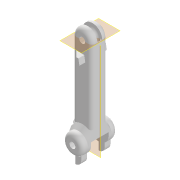
# Autodesk Inventor part: index_f1
Saved by Autodesk Inventor 2020.2 (Build 242310000, 310)
## iProperties
Created: 2020-04-08
Part Number: index_f1
Material: Generic
Document SubType Name: Modeling
Designer: Bardo91
Density: 1 g/cm^3
Appearance: Default
Author: Bardo91
Autodesk Inventor part; units mm, degrees
ref_plane "YZ Plane" through (0, 0, 0) normal (1, 0, 0) x (0, 1, 0)
ref_plane "XY Plane" through (0, 0, 0) normal (0, 0, 1) x (1, 0, 0)
sketch "Sketch1" plane through (0, 0, 0) normal (0, 0, 1) x (1, 0, 0)
  circle A0 centre (0, 0) radius 1.5
  line L0 (0, 0) -> (0, 44)
  circle A1 centre (0, 44) radius 1.5
  circle A2 centre (0, 44) radius 5
  circle A3 centre (0, 0) radius 5
  line L1 (-5, 44) -> (-5, 0)
  line L2 (5, 0) -> (5, 44)
  point P0 (0, 39)
  point P1 (0, 5)
  dimension "d0" = 3
  dimension "d1" = 44
  dimension "d2" = 3
  dimension "d3" = 10
  dimension "d4" = 10
  constraints: 6 end point, 4 centre point, 4 coincident, 4 point on circle, 2 tangent, 2 vertical
  measures "d0" diameter of A0
  measures "d1" distance of L0.start L0.end
  measures "d2" diameter of A1
  measures "d3" diameter of A2
  measures "d4" diameter of A3
extrude "base" add sketch "Sketch1" along normal blind 8
sketch "Sketch2" plane through (0, 0, 8) normal (0, 0, 1) x (1, 0, 0)
  circle A0 centre (0, 0) radius 1.5 projected
  circle A1 centre (0, 0) radius 5
  circle A2 centre (0, 0) radius 1.5
  dimension "d7" = 10
  dimension "d8" = 3
  constraints: 2 centre point, 2 coincident
  measures "d7" diameter of A1
  measures "d8" diameter of A2
extrude "joint" add sketch "Sketch2" along normal blind 5
ref_plane "Work Plane1" through (0, 0, 4) normal (0, 0, 1) x (1, 0, 0)
mirror "Mirror1" about plane through (0, 0, 4) normal (0, 0, 1) of "joint"
chamfer "Chamfer1" distance 2 angle 45 2 edges at (0, 5, 8) (0, 5, 0)
sketch "Sketch3" plane through (0, 0, 4) normal (0, 0, 1) x (1, 0, 0)
  circle A0 centre (0, 0) radius 5.25
  circle A1 centre (0, 0) radius 1.5
  line L0 (0, 0.1787) -> (-5.25, 0)
  line L1 (-5.25, 0) -> (-5.25, 4)
  line L2 (-5.25, 0) -> (-1.25, 0) construction
  line L3 (-5.25, 4) -> (0, 0)
  line L4 (0, 5.25) -> (-8.7104, 5.25)
  line L5 (-8.7104, 5.25) -> (-8.7104, 0)
  line L6 (-8.7104, 0) -> (-5.25, 0)
  point P0 (-4.176, 3.1817)
  dimension "d12" = 10.5
  dimension "d13" = 3
  dimension "d45" = 4
  dimension "d46" = 90
  constraints: 14 end point, 3 perpendicular, 2 centre point, 2 coincident, 2 horizontal, 2 point on circle, 1 tangent, 1 vertical
  measures "d12" diameter of A0
  measures "d13" diameter of A1
  measures "d45" distance of L0.end L1.end
  measures "d46" angle of L2 L1
extrude "joint_2" cut sketch "Sketch3" along normal mid plane 9 contours A0 L0 A1 L3 | A0 L3 L1 L6 L5 L4 | L1 L3 A0 | A0 L3 A1 L0
fillet "Fillet2" radius 2 8 edges at (-5, 0, 13) (-5, 0, -5) (-5, 24.625, 0) (5, 24.4495, 0) (0, 49, 0) (0, 49, 8) (-5, 24.625, 8) (5, 24.4495, 8)
sketch "Sketch4" plane through (0, 0, 0) normal (0, 1, 0) x (-1, 0, 0)
  line L0 (-1.5, 8.5) -> (1.5, 8.5) projected
  line L1 (0, 8.5) -> (0, -0.4996)
  line L2 (0, 4.0002) -> (-3.5, 4.0002)
  line L3 (0, 4.0002) -> (3.5, 4.0002)
  circle A0 centre (-3.5, 4.0002) radius 1.25
  circle A1 centre (3.5, 4.0002) radius 1.25
  point P0 (0, 0)
  dimension "d20" = 3.5
  dimension "d21" = 3.5
  dimension "thread_hole" = 2.5
  dimension "d23" = 2.5
  constraints: 6 end point, 2 centre point, 2 coincident, 2 horizontal, 2 midpoint, 1 vertical
  measures "d20" distance of L2.start L2.end
  measures "d21" distance of L2.start L3.end
  measures "thread_hole" diameter of A0
  measures "d23" diameter of A1
extrude "thread_hole" cut sketch "Sketch4" along normal through all contours A0
ref_plane "Work Plane2" through (5, 44, 2) normal (0, 1, 0) x (-1, 0, 0)
sketch "Sketch9" plane through (5, 44, 2) normal (0, 1, 0) x (-1, 0, 0)
  line L0 (5, -2) -> (5, 6)
  line L1 (8, 6) -> (2, 6) projected
  line L2 (5, 2) -> (1.5, 2)
  circle A0 centre (1.5, 2) radius 1.25
  line L3 (1.5, 0.75) -> (0, 0.75)
  line L4 (0, 0) -> (0, 4) projected
  line L5 (1.5, 3.25) -> (0, 3.25)
  dimension "d47" = 3.5
  dimension "d48" = 2.5
  constraints: 8 end point, 2 horizontal, 2 midpoint, 2 point on circle, 2 point on line, 1 centre point, 1 coincident, 1 parallel, 1 tangent
  measures "d47" distance of L2.start L2.end
  measures "d48" diameter of A0
revolve "Revolution2" cut sketch "Sketch9" angle 180 about axis through (0, 44, 0) along (0, 0, 1)
sketch "Sketch10" plane through (-5, 44, 2.75) normal (0, 1, 0) x (1, 0, 0)
  arc A0 (1.5, -2.5) -> (1.5, 0) centre (1.5, -1.25) ccw projected
  circle A1 centre (1.5, -1.25) radius 1.25
  point P0 (5, 2.75)
  constraints: 1 coincident, 3 other
extrude "Extrusion8" cut sketch "Sketch10" against normal through all
sketch "Sketch11" plane through (0, 0, 8.5) normal (0, 0, -1) x (-1, 0, 0)
  line L0 (0, 0) -> (0, -5)
  arc A0 (-5, 0) -> (5, 0) centre (0, 0) ccw projected
  line L1 (0, -5) -> (0, -9)
  line L2 (0, -9) -> (-3, -9)
  line L3 (-3, -9) -> (-3, -4)
  dimension "d52" = 4
  dimension "d53" = 3
  constraints: 8 end point, 2 perpendicular, 2 point on circle, 1 point on line, 1 vertical
  measures "d52" distance of L0.end L1.end
  measures "d53" distance of L1.end L2.end
extrude "Extrusion9" add sketch "Sketch11" against normal blind 3
mirror "Mirror4" about plane through (0, 0, 4) normal (0, 0, 1) of "Extrusion9"
fillet "Fillet4" radius 3 2 edges at (3, -9, 10) (3, -9, -2)
sketch "Sketch12" plane through (0, 0, 8) normal (0, 0, 1) x (1, 0, 0)
  circle A0 centre (0, 44) radius 1.5 projected
  line L0 (0, 44) -> (0, 38)
  line L1 (0, 38) -> (0, 35)
  line L2 (0, 44) -> (1.5869, 35)
  line L3 (0, 44) -> (9.1388, 44) construction
  line L4 (1.5869, 35) -> (0, 35)
  line L5 (2.25, 4.7434) -> (2.25, 44.0003) projected
  line L6 (0, 38) -> (1.058, 38)
  point P0 (0, 0)
  dimension "d57" = 6
  dimension "d58" = 3
  dimension "d59" = 80
  constraints: 12 end point, 2 point on line, 1 equal length, 1 horizontal, 1 parallel, 1 perpendicular, 1 vertical
  measures "d57" distance of L0.start L0.end
  measures "d58" distance of L0.end L1.end
  measures "d59" angle of L2 L3
extrude "Extrusion10" add sketch "Sketch12" along normal blind 3 contours L6 L2 L4 L1
mirror "Mirror5" about plane through (0, 0, 4) normal (0, 0, 1) of "Extrusion10"
chamfer "Chamfer3" distance 3 angle 45 2 edges at (0, 36.5, 8) (0, 36.5, 0)
sketch "Sketch7" plane through (0, 0, 8) normal (0, 0, 1) x (1, 0, 0)
  circle A0 centre (0, 44) radius 1.5 projected
  line L0 (0, 44) -> (-1.0419, 49.9088)
  line L1 (0, 44) -> (6, 44) construction
  line L2 (-1.0419, 49.9088) -> (-0.1736, 44.9848)
  line L3 (0, 44) -> (0, 44.9848)
  line L4 (0, 44.9848) -> (-0.1736, 44.9848)
  line L5 (-1.0419, 49.9088) -> (0, 49.9088)
  point P0 (0, 0)
  dimension "d32" = 6
  dimension "d33" = 80
  dimension "d34" = 5
  constraints: 12 end point, 2 perpendicular, 2 point on line, 1 equal length, 1 horizontal, 1 vertical
  measures "d32" distance of L0.start L0.end
  measures "d33" angle of L0 L1
  measures "d34" distance of L0.end L2.end
sketch "Sketch8" plane through (0, 0, 8.5) normal (0, 0, -1) x (-1, 0, 0)
  line L0 (0, 0) -> (0, -5)
  arc A0 (-5, 0) -> (5, 0) centre (0, 0) ccw projected
  line L1 (0, -5) -> (0, -9)
  line L2 (0, -9) -> (-3, -9)
  line L3 (-3, -9) -> (-3, -4)
  dimension "d40" = 4
  dimension "d41" = 3
  constraints: 8 end point, 2 point on circle, 1 horizontal, 1 perpendicular, 1 point on line, 1 vertical
  measures "d40" distance of L0.end L1.end
  measures "d41" distance of L1.end L2.end
equation "\"d23\" = thread_hole"
equation "\"d48\" = thread_hole"
body "Solid1"
